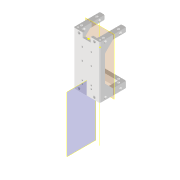
# Autodesk Inventor part: 30_Linear_Stage_NEMA11_China_base_universal_v3
Saved by Autodesk Inventor 2022 (Build 260153000, 153)
## iProperties
Created: 2022-02-11
Part Number: 30_Linear_Stage_NEMA11_China_base_universal_v3
Material: Generic
Document SubType Name: Modeling
Designer: wanghaoran
Density: 1 g/cm^3
Appearance: Default
Catalog Web Link: isPrinted
Vendor: openUC2
Mass: 36.1859 g
Surface Area: 194.638 cm^2
Volume: 36.1859 cm^3
Author: wanghaoran
Autodesk Inventor part; units mm, degrees
note: some values were not read from the file. Chosen so that the rebuilt part matches the saved one: pattern direction of "Runde Anordnung2".
ref_plane "YZ Plane" through (0, 0, 0) normal (1, 0, 0) x (0, 1, 0)
ref_plane "XZ Plane" through (0, 0, 0) normal (0, 1, 0) x (-1, 0, 0)
sketch "Sketch1" plane through (0, 0, 0) normal (0, 1, 0) x (-1, 0, 0)
  line L0 (0, 0) -> (49.8, 0)
  line L1 (49.8, 0) -> (49.8, -49.8)
  line L2 (49.8, -49.8) -> (0, -49.8)
  line L3 (0, -49.8) -> (0, 0)
  line L4 (7.8, -7.8) -> (42, -7.8)
  line L5 (42, -7.8) -> (42, -42)
  line L6 (42, -42) -> (7.8, -42)
  line L7 (7.8, -42) -> (7.8, -7.8)
  line L8 (39.9, -4.55) -> (9.9, -4.55) projected
  line L9 (42, -7.8) -> (7.8, -7.8)
  line L10 (7.8, -7.8) -> (7.8, -4.55)
  line L11 (7.8, -4.55) -> (42, -4.55)
  line L12 (42, -4.55) -> (42, -7.8)
  dimension "d0" = 49.8
  dimension "d1" = 49.8
  dimension "d2" = 7.8
  constraints: 24 end point, 6 parallel, 3 perpendicular, 2 horizontal, 3 other
  measures "d0" distance of L1.end L2.end
  measures "d1" distance of L0.end L1.end
  measures "d2" distance between parallel lines of L3 L7
extrude "Extrusion1" add sketch "Sketch1" along normal blind 12
sketch "Sketch3" plane through (0, 0, 0) normal (0, -1, 0) x (1, 0, 0)
  line L0 (-49.8, 0) -> (0, 0) projected
  line L1 (-49.8, -49.8) -> (-49.8, 0) projected
  line L2 (0, 0) -> (-49.8, 0)
  line L3 (-49.8, 0) -> (-49.8, -4.55)
  line L4 (-49.8, -4.55) -> (0, -4.55)
  line L5 (0, -4.55) -> (0, 0)
  line L6 (-7.8, -42) -> (-7.8, -4.55) projected
  line L7 (0, -49.8) -> (-7.8, -49.8)
  line L8 (-7.8, -49.8) -> (-7.8, -42)
  line L9 (-7.8, -42) -> (0, -42)
  line L10 (0, -42) -> (0, -49.8)
  line L11 (0, -49.8) -> (-49.8, -49.8) projected
  line L12 (-42, -4.55) -> (-42, -42) projected
  line L13 (-49.8, -49.8) -> (-42, -49.8)
  line L14 (-42, -49.8) -> (-42, -42)
  line L15 (-42, -42) -> (-49.8, -42)
  line L16 (-49.8, -42) -> (-49.8, -49.8)
  line L17 (-7.8, -4.55) -> (-42, -4.55) projected
  line L18 (-49.8, -4.55) -> (-42, -4.55)
  line L19 (-42, -4.55) -> (-42, -10)
  line L20 (-42, -10) -> (-49.8, -10)
  line L21 (-49.8, -10) -> (-49.8, -4.55)
  line L22 (0, -4.55) -> (-7.8, -4.55)
  line L23 (-7.8, -4.55) -> (-7.8, -10)
  line L24 (-7.8, -10) -> (0, -10)
  line L25 (0, -10) -> (0, -4.55)
  point P0 (-7.8, -7.8)
  point P1 (-42, -7.8)
  point P2 (-7.8, -7.8)
  point P3 (-42, -7.8)
  dimension "d57" = 0
  dimension "d58" = 10
  dimension "d59" = 10
  constraints: 40 end point, 10 parallel, 5 horizontal, 5 perpendicular, 3 point on line
  measures "d57" distance between parallel lines of L17 L4
  measures "d58" distance between parallel lines of L20 L0
  measures "d59" distance between parallel lines of L24 L0
extrude "Extrusion2" add sketch "Sketch3" against normal blind 92 contours L0 L5 L4 L1 | L4 L12 L20 L1 | L25 L24 L6 L4
sketch "Sketch4" plane through (-49.8, 0, 0) normal (0, 0, 1) x (1, 0, 0)
  line L0 (23.45, 81) -> (26.35, 81)
  line L1 (26.35, 81) -> (26.35, 11)
  line L2 (26.35, 11) -> (23.45, 11)
  line L3 (23.45, 11) -> (23.45, 81)
  line L4 (49.8, 0) -> (49.8, 92) projected
  line L5 (0, 0) -> (49.8, 0) projected
  circle A0 centre (24.9, 81) radius 1.45
  circle A1 centre (24.9, 11) radius 1.45
  line L6 (0, 92) -> (49.8, 92) projected
  circle A2 centre (33.4, 21) radius 1.45
  circle A3 centre (16.4, 21) radius 1.45
  circle A4 centre (33.4, 76) radius 1.45
  circle A5 centre (16.4, 76) radius 1.45
  line L7 (-75.7089, 93.7838) -> (-35.7089, 93.7838)
  line L8 (-35.7089, 93.7838) -> (-35.7089, -0.2162)
  line L9 (-35.7089, -0.2162) -> (-75.7089, -0.2162)
  line L10 (-75.7089, -0.2162) -> (-75.7089, 93.7838)
  circle A6 centre (-67.7652, 52.7838) radius 1.45
  circle A7 centre (-67.7652, 14.7838) radius 1.45
  circle A8 centre (16.4, 15) radius 1.45
  circle A9 centre (33.4, 15) radius 1.45
  circle A10 centre (16.4, 53) radius 1.45
  circle A11 centre (33.4, 53) radius 1.45
  dimension "d9" = 2.9
  dimension "d10" = 70
  dimension "d11" = 23.45
  dimension "d12" = 11
  dimension "d123" = 2.9
  dimension "d125" = 21
  dimension "d128" = 7.05
  dimension "d131" = 17
  dimension "d134" = 55
  dimension "d155" = 40
  dimension "d156" = 94
  dimension "d157" = 2.9
  dimension "d161" = 38
  dimension "d166" = 15
  dimension "d167" = 2.9
  dimension "d168" = 2.9
  dimension "d169" = 15
  dimension "d170" = 15
  dimension "d173" = 38
  constraints: 16 end point, 10 centre point, 4 parallel, 3 horizontal, 3 vertical, 2 midpoint, 2 perpendicular, 18 other
  measures "d9" distance of L1.end L2.end
  measures "d10" distance of L0.end L1.end
  measures "d11" distance between parallel lines of L4 L1
  measures "d12" distance between parallel lines of L5 L2
  measures "d123" diameter of A2
  measures "d125" distance from line of L5 A2.centre
  measures "d128" distance from line of A2.centre L1
  measures "d131" distance of A2.centre A3.centre
  measures "d134" distance of A2.centre A4.centre
  measures "d155" distance of L8.end L9.end
  measures "d156" distance of L7.end L8.end
  measures "d157" diameter of A6
  measures "d161" distance of A6.centre A7.centre
  measures "d166" distance from line of L9 A7.centre
  measures "d167" diameter of A8
  measures "d168" diameter of A9
  measures "d169" distance from line of L5 A8.centre
  measures "d170" distance from line of L5 A9.centre
  measures "d173" distance of A8.centre A10.centre
extrude "Extrusion3" cut sketch "Sketch4" against normal up to next contours A2 | A3 | A4 | A5 | A8 | A9 | A10 | A11
sketch "Sketch5" plane through (0, 92, 0) normal (0, 1, 0) x (1, 0, 0)
  circle A0 centre (-45.9, 45.9) radius 1.4
  circle A1 centre (-3.9, 45.9) radius 1.4
  line L0 (-49.8, 49.8) -> (-49.8, 0) projected
  line L1 (-49.8, 24.9) -> (-42, 24.9)
  line L2 (-42, 4.55) -> (-42, 42) projected
  line L3 (-49.8, 0) -> (0, 0) projected
  line L4 (0, 0) -> (0, 10) projected
  line L5 (0, 10) -> (-7.8, 10) projected
  line L6 (-7.8, 10) -> (-7.8, 4.55) projected
  line L7 (-49.8, 10) -> (-49.8, 0) projected
  line L8 (0, 49.8) -> (-49.8, 49.8) projected
  line L9 (-49.8, 0) -> (0, 0)
  line L10 (0, 0) -> (0, 49.8)
  line L11 (0, 49.8) -> (-49.8, 49.8)
  line L12 (-49.8, 49.8) -> (-49.8, 0)
  circle A2 centre (-4.9, 4.9) radius 2.4
  circle A3 centre (-44.9, 4.9) radius 2.4
  circle A4 centre (-4.9, 4.9) radius 1.4
  circle A5 centre (-44.9, 4.9) radius 1.4
  line L13 (-7.8, 4.55) -> (-42, 4.55) projected
  line L14 (-42, 4.55) -> (-42, 10) projected
  line L15 (-42, 10) -> (-49.8, 10) projected
  point P0 (-42, 7.8)
  dimension "d28" = 2.8
  dimension "d29" = 2.8
  dimension "d90" = 2.8
  dimension "d91" = 2.8
  dimension "d92" = 40
  dimension "d93" = 4.9
  dimension "d94" = 4.9
  dimension "d95" = 4.9
  constraints: 10 end point, 6 centre point, 2 coincident, 2 horizontal, 2 parallel, 1 midpoint, 1 perpendicular, 1 point on line
  measures "d28" diameter of A0
  measures "d29" diameter of A1
  measures "d90" diameter of A4
  measures "d91" diameter of A5
  measures "d92" distance of A4.centre A5.centre
  measures "d93" distance from line of L12 A5.centre
  measures "d94" distance from line of L3 A5.centre
  measures "d95" distance from line of L9 A2.centre
extrude "Extrusion4" cut sketch "Sketch5" against normal blind 20 contours A0 | A1 | A4 | A5
fillet "Fillet1" radius 2 4 edges at (0, 46, 0) (0, 6, -49.8) (-49.8, 6, -49.8) (-49.8, 46, 0)
ref_plane "Arbeitsebene1" through (-24.9, 12, -4.55) normal (-1, 0, 0) x (0, 0, -1)
ref_plane "Arbeitsebene2" through (-47.8, 0, -24.9) normal (0, 0, 1) x (1, 0, 0)
sketch "Skizze8" plane through (0, 0, 0) normal (0, -1, 0) x (1, 0, 0)
  line L0 (-49.9, -29.9) -> (-49.9, -47.9) projected
  arc A0 (-49.9, -47.9) -> (-47.9, -49.9) centre (-47.9, -47.9) ccw projected
  line L1 (-30.0511, -49.9) -> (-47.9, -49.9) projected
  line L2 (-30.0511, -49.9) -> (-30.0509, -49.1742) projected
  arc A1 (-30.0509, -49.1742) -> (-30.2806, -48.8498) centre (-30.3999, -49.1778) ccw projected
  arc A2 (-31.9947, -46.7407) -> (-30.2806, -48.8498) centre (-29.84, -46.7407) ccw projected
  line L3 (-31.9947, -46.7407) -> (-31.9947, -46.6009) projected
  arc A3 (-29.8434, -44.4498) -> (-31.9947, -46.6009) centre (-29.8435, -46.6009) ccw projected
  line L4 (-29.8434, -44.4498) -> (-19.9598, -44.4503) projected
  arc A4 (-17.81, -46.6004) -> (-19.9598, -44.4503) centre (-19.96, -46.6003) ccw projected
  line L5 (-17.81, -46.6004) -> (-17.81, -46.7408) projected
  arc A5 (-19.52, -48.8451) -> (-17.81, -46.7408) centre (-19.9599, -46.7406) ccw projected
  arc A6 (-19.52, -48.8451) -> (-19.7498, -49.1739) centre (-19.3996, -49.1739) ccw projected
  line L6 (-19.7498, -49.1739) -> (-19.7495, -49.9) projected
  line L7 (-1.9, -49.9) -> (-19.7495, -49.9) projected
  arc A7 (-1.9, -49.9) -> (0.1, -47.9) centre (-1.9, -47.9) ccw projected
  line L8 (0.1, -47.9) -> (0.1, -30.0511) projected
  line L9 (0.1, -30.0511) -> (-0.6258, -30.0509) projected
  arc A8 (-0.6258, -30.0509) -> (-0.9502, -30.2806) centre (-0.6222, -30.3999) ccw projected
  arc A9 (-3.0593, -31.9947) -> (-0.9502, -30.2806) centre (-3.0593, -29.84) ccw projected
  line L10 (-3.0593, -31.9947) -> (-3.1991, -31.9947) projected
  arc A10 (-5.3502, -29.8434) -> (-3.1991, -31.9947) centre (-3.1991, -29.8435) ccw projected
  line L11 (-5.3502, -29.8434) -> (-5.3497, -19.9598) projected
  arc A11 (-3.1996, -17.81) -> (-5.3497, -19.9598) centre (-3.1997, -19.96) ccw projected
  line L12 (-3.1996, -17.81) -> (-3.0592, -17.81) projected
  arc A12 (-0.9549, -19.52) -> (-3.0592, -17.81) centre (-3.0594, -19.9599) ccw projected
  arc A13 (-0.9549, -19.52) -> (-0.6261, -19.7498) centre (-0.6261, -19.3996) ccw projected
  line L13 (-0.6261, -19.7498) -> (0.1, -19.7495) projected
  line L14 (0.1, -19.7495) -> (0.1, -1.9) projected
  arc A14 (0.1, -1.9) -> (-1.9, 0.1) centre (-1.9, -1.9) ccw projected
  line L15 (-19.9, 0.1) -> (-1.9, 0.1) projected
  line L16 (-19.9, 0.1) -> (-19.9, 0.9263) projected
  arc A15 (-19.56, 1.4) -> (-19.9, 0.9263) centre (-19.4, 0.9263) ccw projected
  arc A16 (-19.56, 1.4) -> (-17.96, 3.3596) centre (-19.96, 3.3596) ccw projected
  line L17 (-17.96, 3.3596) -> (-17.96, 3.5) projected
  arc A17 (-17.96, 3.5) -> (-19.96, 5.5) centre (-19.96, 3.5) ccw projected
  line L18 (-19.96, 5.5) -> (-29.84, 5.5) projected
  arc A18 (-29.84, 5.5) -> (-31.84, 3.5) centre (-29.84, 3.5) ccw projected
  line L19 (-31.84, 3.5) -> (-31.84, 3.3596) projected
  arc A19 (-31.84, 3.3596) -> (-30.24, 1.4) centre (-29.84, 3.3596) ccw projected
  arc A20 (-29.9, 0.9263) -> (-30.24, 1.4) centre (-30.4, 0.9263) ccw projected
  line L20 (-29.9, 0.9263) -> (-29.9, 0.1) projected
  line L21 (-47.9, 0.1) -> (-29.9, 0.1) projected
  arc A21 (-47.9, 0.1) -> (-49.9, -1.9) centre (-47.9, -1.9) ccw projected
  line L22 (-49.9, -1.9) -> (-49.9, -19.9) projected
  line L23 (-49.9, -19.9) -> (-50.7263, -19.9) projected
  arc A22 (-51.2, -19.56) -> (-50.7263, -19.9) centre (-50.7263, -19.4) ccw projected
  arc A23 (-51.2, -19.56) -> (-53.1596, -17.96) centre (-53.1596, -19.96) ccw projected
  line L24 (-53.1596, -17.96) -> (-53.3, -17.96) projected
  arc A24 (-53.3, -17.96) -> (-55.3, -19.96) centre (-53.3, -19.96) ccw projected
  line L25 (-55.3, -19.96) -> (-55.3, -29.84) projected
  arc A25 (-55.3, -29.84) -> (-53.3, -31.84) centre (-53.3, -29.84) ccw projected
  line L26 (-53.3, -31.84) -> (-53.1596, -31.84) projected
  arc A26 (-53.1596, -31.84) -> (-51.2, -30.24) centre (-53.1596, -29.84) ccw projected
  arc A27 (-50.7263, -29.9) -> (-51.2, -30.24) centre (-50.7263, -30.4) ccw projected
  line L27 (-50.7263, -29.9) -> (-49.9, -29.9) projected
  arc A28 (-49.9, -26.2329) -> (-49.9, -23.7671) centre (-46.2, -25) ccw projected
  line L28 (-49.9, -26.2329) -> (-49.9, -23.7671) projected
  circle A29 centre (-25, -3.6) radius 3.9 projected
  line L29 (-7.6, -40.2) -> (-7.6, -9.6) projected
  arc A30 (-9.6, -42.2) -> (-7.6, -40.2) centre (-9.6, -40.2) ccw projected
  line L30 (-9.6, -42.2) -> (-40.2, -42.2) projected
  arc A31 (-42.2, -40.2) -> (-40.2, -42.2) centre (-40.2, -40.2) ccw projected
  line L31 (-42.2, -9.6) -> (-42.2, -40.2) projected
  arc A32 (-40.2, -7.6) -> (-42.2, -9.6) centre (-40.2, -9.6) ccw projected
  line L32 (-40.2, -7.6) -> (-9.6, -7.6) projected
  arc A33 (-7.6, -9.6) -> (-9.6, -7.6) centre (-9.6, -9.6) ccw projected
  circle A34 centre (-44.8, -5) radius 2.4 projected
  circle A35 centre (-39.35, -4.35) radius 2.45 projected
  circle A36 centre (-45.45, -10.45) radius 2.45 projected
  circle A37 centre (-4.35, -10.45) radius 2.45 projected
  circle A38 centre (-10.45, -4.35) radius 2.45 projected
  circle A39 centre (-5, -5) radius 2.4 projected
  circle A40 centre (-45.45, -39.35) radius 2.45 projected
  circle A41 centre (-39.35, -45.45) radius 2.45 projected
  circle A42 centre (-44.8, -44.8) radius 2.4 projected
  circle A43 centre (-4.35, -39.35) radius 2.45 projected
  circle A44 centre (-10.45, -45.45) radius 2.45 projected
  circle A45 centre (-5, -44.8) radius 2.4 projected
  point P0 (0, 0)
hole "Bohrung1" at (-45.45, 0, -39.35) at (-39.35, 0, -4.35) at (-10.45, 0, -4.35) at (-4.35, 0, -39.35) at (-10.45, 0, -45.45) at (-39.35, 0, -45.45) direction (0, 1, 0) diameter 4.8 depth 12 tip angle 118
sketch "Skizze10" plane through (0, 92, 0) normal (0, 1, 0) x (1, 0, 0)
  arc A0 (-25.6984, 4.55) -> (-24.1016, 4.55) centre (-24.9, 3.4) ccw projected
  point P0 (0, 0)
sketch "Skizze11" plane through (-47.8, 0, 0) normal (0, 0, 1) x (1, 0, 0)
  line L0 (7.74, 57.65) -> (37.74, 57.65) projected
  arc A0 (5.24, 60.15) -> (7.74, 57.65) centre (7.74, 60.15) ccw projected
  line L1 (5.24, 90.15) -> (5.24, 60.15) projected
  arc A1 (7.74, 92.65) -> (5.24, 90.15) centre (7.74, 90.15) ccw projected
  line L2 (37.74, 92.65) -> (7.74, 92.65) projected
  arc A2 (40.24, 90.15) -> (37.74, 92.65) centre (37.74, 90.15) ccw projected
  line L3 (40.24, 60.15) -> (40.24, 90.15) projected
  arc A3 (37.74, 57.65) -> (40.24, 60.15) centre (37.74, 60.15) ccw projected
  circle A4 centre (22.74, 53.15) radius 4 projected
  line L4 (40.99, 91.1222) -> (43.54, 92.5945) projected
  line L5 (43.54, 92.5945) -> (46.09, 91.1222) projected
  line L6 (46.09, 91.1222) -> (46.09, 88.1778) projected
  line L7 (46.09, 88.1778) -> (43.54, 86.7055) projected
  line L8 (43.54, 86.7055) -> (40.99, 88.1778) projected
  line L9 (40.99, 88.1778) -> (40.99, 91.1222) projected
  line L10 (35.7678, 93.4) -> (34.2955, 95.95) projected
  line L11 (34.2955, 95.95) -> (35.7678, 98.5) projected
  line L12 (35.7678, 98.5) -> (38.7122, 98.5) projected
  line L13 (38.7122, 98.5) -> (40.1845, 95.95) projected
  line L14 (40.1845, 95.95) -> (38.7122, 93.4) projected
  line L15 (38.7122, 93.4) -> (35.7678, 93.4) projected
  line L16 (40.99, 59.1778) -> (43.54, 57.7055) projected
  line L17 (40.99, 62.1222) -> (40.99, 59.1778) projected
  line L18 (43.54, 63.5945) -> (40.99, 62.1222) projected
  line L19 (46.09, 62.1222) -> (43.54, 63.5945) projected
  line L20 (46.09, 59.1778) -> (46.09, 62.1222) projected
  line L21 (43.54, 57.7055) -> (46.09, 59.1778) projected
  line L22 (35.7678, 56.9) -> (34.2955, 54.35) projected
  line L23 (38.7122, 56.9) -> (35.7678, 56.9) projected
  line L24 (40.1845, 54.35) -> (38.7122, 56.9) projected
  line L25 (38.7122, 51.8) -> (40.1845, 54.35) projected
  line L26 (35.7678, 51.8) -> (38.7122, 51.8) projected
  line L27 (34.2955, 54.35) -> (35.7678, 51.8) projected
  line L28 (4.49, 91.1222) -> (1.94, 92.5945) projected
  line L29 (4.49, 88.1778) -> (4.49, 91.1222) projected
  line L30 (1.94, 86.7055) -> (4.49, 88.1778) projected
  line L31 (-0.61, 88.1778) -> (1.94, 86.7055) projected
  line L32 (-0.61, 91.1222) -> (-0.61, 88.1778) projected
  line L33 (1.94, 92.5945) -> (-0.61, 91.1222) projected
  line L34 (9.7122, 93.4) -> (11.1845, 95.95) projected
  line L35 (6.7678, 93.4) -> (9.7122, 93.4) projected
  line L36 (5.2955, 95.95) -> (6.7678, 93.4) projected
  line L37 (6.7678, 98.5) -> (5.2955, 95.95) projected
  line L38 (9.7122, 98.5) -> (6.7678, 98.5) projected
  line L39 (11.1845, 95.95) -> (9.7122, 98.5) projected
  line L40 (9.7122, 56.9) -> (11.1845, 54.35) projected
  line L41 (11.1845, 54.35) -> (9.7122, 51.8) projected
  line L42 (9.7122, 51.8) -> (6.7678, 51.8) projected
  line L43 (6.7678, 51.8) -> (5.2955, 54.35) projected
  line L44 (5.2955, 54.35) -> (6.7678, 56.9) projected
  line L45 (6.7678, 56.9) -> (9.7122, 56.9) projected
  line L46 (4.49, 59.1778) -> (1.94, 57.7055) projected
  line L47 (1.94, 57.7055) -> (-0.61, 59.1778) projected
  line L48 (-0.61, 59.1778) -> (-0.61, 62.1222) projected
  line L49 (-0.61, 62.1222) -> (1.94, 63.5945) projected
  line L50 (1.94, 63.5945) -> (4.49, 62.1222) projected
  line L51 (4.49, 62.1222) -> (4.49, 59.1778) projected
  circle A5 centre (0.74, 75.15) radius 4 projected
  line L52 (46.8233, 69.2502) -> (47.24, 69.2503) projected
  arc A6 (41.54, 70.1) -> (46.8233, 69.2502) centre (44.25, 70.1) ccw projected
  line L53 (41.54, 80.2) -> (41.54, 70.1) projected
  arc A7 (46.8233, 81.0498) -> (41.54, 80.2) centre (44.25, 80.2) ccw projected
  line L54 (47.24, 81.0497) -> (46.8233, 81.0498) projected
  line L55 (47.24, 98.15) -> (47.24, 81.0497) projected
  arc A8 (47.24, 98.15) -> (45.74, 99.65) centre (45.74, 98.15) ccw projected
  line L56 (28.6397, 99.65) -> (45.74, 99.65) projected
  line L57 (28.6398, 99.2333) -> (28.6397, 99.65) projected
  arc A9 (27.79, 93.95) -> (28.6398, 99.2333) centre (27.79, 96.66) ccw projected
  line L58 (17.69, 93.95) -> (27.79, 93.95) projected
  arc A10 (16.8402, 99.2333) -> (17.69, 93.95) centre (17.69, 96.66) ccw projected
  line L59 (16.8403, 99.65) -> (16.8402, 99.2333) projected
  line L60 (-0.26, 99.65) -> (16.8403, 99.65) projected
  arc A11 (-0.26, 99.65) -> (-1.76, 98.15) centre (-0.26, 98.15) ccw projected
  line L61 (-1.76, 79.65) -> (-1.76, 98.15) projected
  line L62 (-3.6239, 79.65) -> (-1.76, 79.65) projected
  arc A12 (-4.3693, 80.3167) -> (-3.6239, 79.65) centre (-3.6239, 80.4) ccw projected
  arc A13 (-4.3693, 80.3167) -> (-7.36, 80.15) centre (-5.86, 80.15) ccw projected
  line L63 (-7.36, 70.15) -> (-7.36, 80.15) projected
  arc A14 (-7.36, 70.15) -> (-4.3693, 69.9833) centre (-5.86, 70.15) ccw projected
  arc A15 (-3.6239, 70.65) -> (-4.3693, 69.9833) centre (-3.6239, 69.9) ccw projected
  line L64 (-1.76, 70.65) -> (-3.6239, 70.65) projected
  line L65 (-1.76, 52.15) -> (-1.76, 70.65) projected
  arc A16 (-1.76, 52.15) -> (-0.26, 50.65) centre (-0.26, 52.15) ccw projected
  line L66 (18.24, 50.65) -> (-0.26, 50.65) projected
  line L67 (18.24, 48.7861) -> (18.24, 50.65) projected
  arc A17 (17.5733, 48.0407) -> (18.24, 48.7861) centre (17.49, 48.7861) ccw projected
  arc A18 (17.5733, 48.0407) -> (17.74, 45.05) centre (17.74, 46.55) ccw projected
  line L68 (27.74, 45.05) -> (17.74, 45.05) projected
  arc A19 (27.74, 45.05) -> (27.9067, 48.0407) centre (27.74, 46.55) ccw projected
  arc A20 (27.24, 48.7861) -> (27.9067, 48.0407) centre (27.99, 48.7861) ccw projected
  line L69 (27.24, 50.65) -> (27.24, 48.7861) projected
  line L70 (45.74, 50.65) -> (27.24, 50.65) projected
  arc A21 (45.74, 50.65) -> (47.24, 52.15) centre (45.74, 52.15) ccw projected
  line L71 (47.24, 69.2503) -> (47.24, 52.15) projected
  line L72 (7.74, 7.65) -> (37.74, 7.65) projected
  arc A22 (5.24, 10.15) -> (7.74, 7.65) centre (7.74, 10.15) ccw projected
  line L73 (5.24, 40.15) -> (5.24, 10.15) projected
  arc A23 (7.74, 42.65) -> (5.24, 40.15) centre (7.74, 40.15) ccw projected
  line L74 (37.74, 42.65) -> (7.74, 42.65) projected
  arc A24 (40.24, 40.15) -> (37.74, 42.65) centre (37.74, 40.15) ccw projected
  line L75 (40.24, 10.15) -> (40.24, 40.15) projected
  arc A25 (37.74, 7.65) -> (40.24, 10.15) centre (37.74, 10.15) ccw projected
  circle A26 centre (22.74, 3.15) radius 4 projected
  line L76 (40.99, 41.1222) -> (43.54, 42.5945) projected
  line L77 (43.54, 42.5945) -> (46.09, 41.1222) projected
  line L78 (46.09, 41.1222) -> (46.09, 38.1778) projected
  line L79 (46.09, 38.1778) -> (43.54, 36.7055) projected
  line L80 (43.54, 36.7055) -> (40.99, 38.1778) projected
  line L81 (40.99, 38.1778) -> (40.99, 41.1222) projected
  line L82 (35.7678, 43.4) -> (34.2955, 45.95) projected
  line L83 (34.2955, 45.95) -> (35.7678, 48.5) projected
  line L84 (35.7678, 48.5) -> (38.7122, 48.5) projected
  line L85 (38.7122, 48.5) -> (40.1845, 45.95) projected
  line L86 (40.1845, 45.95) -> (38.7122, 43.4) projected
  line L87 (38.7122, 43.4) -> (35.7678, 43.4) projected
  line L88 (40.99, 9.1778) -> (43.54, 7.7055) projected
  line L89 (40.99, 12.1222) -> (40.99, 9.1778) projected
  line L90 (43.54, 13.5945) -> (40.99, 12.1222) projected
  line L91 (46.09, 12.1222) -> (43.54, 13.5945) projected
  line L92 (46.09, 9.1778) -> (46.09, 12.1222) projected
  line L93 (43.54, 7.7055) -> (46.09, 9.1778) projected
  line L94 (35.7678, 6.9) -> (34.2955, 4.35) projected
  line L95 (38.7122, 6.9) -> (35.7678, 6.9) projected
  line L96 (40.1845, 4.35) -> (38.7122, 6.9) projected
  line L97 (38.7122, 1.8) -> (40.1845, 4.35) projected
  line L98 (35.7678, 1.8) -> (38.7122, 1.8) projected
  line L99 (34.2955, 4.35) -> (35.7678, 1.8) projected
  line L100 (4.49, 41.1222) -> (1.94, 42.5945) projected
  line L101 (4.49, 38.1778) -> (4.49, 41.1222) projected
  line L102 (1.94, 36.7055) -> (4.49, 38.1778) projected
  line L103 (-0.61, 38.1778) -> (1.94, 36.7055) projected
  line L104 (-0.61, 41.1222) -> (-0.61, 38.1778) projected
  line L105 (1.94, 42.5945) -> (-0.61, 41.1222) projected
  line L106 (9.7122, 43.4) -> (11.1845, 45.95) projected
  line L107 (6.7678, 43.4) -> (9.7122, 43.4) projected
  line L108 (5.2955, 45.95) -> (6.7678, 43.4) projected
  line L109 (6.7678, 48.5) -> (5.2955, 45.95) projected
  line L110 (9.7122, 48.5) -> (6.7678, 48.5) projected
  line L111 (11.1845, 45.95) -> (9.7122, 48.5) projected
  line L112 (9.7122, 6.9) -> (11.1845, 4.35) projected
  line L113 (11.1845, 4.35) -> (9.7122, 1.8) projected
  line L114 (9.7122, 1.8) -> (6.7678, 1.8) projected
  line L115 (6.7678, 1.8) -> (5.2955, 4.35) projected
  line L116 (5.2955, 4.35) -> (6.7678, 6.9) projected
  line L117 (6.7678, 6.9) -> (9.7122, 6.9) projected
  line L118 (4.49, 9.1778) -> (1.94, 7.7055) projected
  line L119 (1.94, 7.7055) -> (-0.61, 9.1778) projected
  line L120 (-0.61, 9.1778) -> (-0.61, 12.1222) projected
  line L121 (-0.61, 12.1222) -> (1.94, 13.5945) projected
  line L122 (1.94, 13.5945) -> (4.49, 12.1222) projected
  line L123 (4.49, 12.1222) -> (4.49, 9.1778) projected
  circle A27 centre (0.74, 25.15) radius 4 projected
  line L124 (46.8233, 19.2502) -> (47.24, 19.2503) projected
  arc A28 (41.54, 20.1) -> (46.8233, 19.2502) centre (44.25, 20.1) ccw projected
  line L125 (41.54, 30.2) -> (41.54, 20.1) projected
  arc A29 (46.8233, 31.0498) -> (41.54, 30.2) centre (44.25, 30.2) ccw projected
  line L126 (47.24, 31.0497) -> (46.8233, 31.0498) projected
  line L127 (47.24, 48.15) -> (47.24, 31.0497) projected
  arc A30 (47.24, 48.15) -> (45.74, 49.65) centre (45.74, 48.15) ccw projected
  line L128 (28.6397, 49.65) -> (45.74, 49.65) projected
  line L129 (28.6398, 49.2333) -> (28.6397, 49.65) projected
  arc A31 (27.79, 43.95) -> (28.6398, 49.2333) centre (27.79, 46.66) ccw projected
  line L130 (17.69, 43.95) -> (27.79, 43.95) projected
  arc A32 (16.8402, 49.2333) -> (17.69, 43.95) centre (17.69, 46.66) ccw projected
  line L131 (16.8403, 49.65) -> (16.8402, 49.2333) projected
  line L132 (-0.26, 49.65) -> (16.8403, 49.65) projected
  arc A33 (-0.26, 49.65) -> (-1.76, 48.15) centre (-0.26, 48.15) ccw projected
  line L133 (-1.76, 29.65) -> (-1.76, 48.15) projected
  line L134 (-3.6239, 29.65) -> (-1.76, 29.65) projected
  arc A34 (-4.3693, 30.3167) -> (-3.6239, 29.65) centre (-3.6239, 30.4) ccw projected
  arc A35 (-4.3693, 30.3167) -> (-7.36, 30.15) centre (-5.86, 30.15) ccw projected
  line L135 (-7.36, 20.15) -> (-7.36, 30.15) projected
  arc A36 (-7.36, 20.15) -> (-4.3693, 19.9833) centre (-5.86, 20.15) ccw projected
  arc A37 (-3.6239, 20.65) -> (-4.3693, 19.9833) centre (-3.6239, 19.9) ccw projected
  line L136 (-1.76, 20.65) -> (-3.6239, 20.65) projected
  line L137 (-1.76, 2.15) -> (-1.76, 20.65) projected
  arc A38 (-1.76, 2.15) -> (-0.26, 0.65) centre (-0.26, 2.15) ccw projected
  line L138 (18.24, 0.65) -> (-0.26, 0.65) projected
  line L139 (18.24, -1.2139) -> (18.24, 0.65) projected
  arc A39 (17.5733, -1.9593) -> (18.24, -1.2139) centre (17.49, -1.2139) ccw projected
  arc A40 (17.5733, -1.9593) -> (17.74, -4.95) centre (17.74, -3.45) ccw projected
  line L140 (27.74, -4.95) -> (17.74, -4.95) projected
  arc A41 (27.74, -4.95) -> (27.9067, -1.9593) centre (27.74, -3.45) ccw projected
  arc A42 (27.24, -1.2139) -> (27.9067, -1.9593) centre (27.99, -1.2139) ccw projected
  line L141 (27.24, 0.65) -> (27.24, -1.2139) projected
  line L142 (45.74, 0.65) -> (27.24, 0.65) projected
  arc A43 (45.74, 0.65) -> (47.24, 2.15) centre (45.74, 2.15) ccw projected
  line L143 (47.24, 19.2503) -> (47.24, 2.15) projected
  point P0 (1.94, 60.65)
  point P1 (43.54, 60.65)
  point P2 (-0.26, 50.15)
  point P3 (45.74, 50.15)
  point P4 (8.24, 4.35)
  point P5 (1.94, 39.65)
  point P6 (37.24, 4.35)
  point P7 (43.54, 39.65)
hole "Bohrung3" at (-39.56, 4.35, 0) at (-10.56, 4.35, 0) direction (0, 0, -1) diameter 4.8 depth 12 tip angle 118
pattern_circular "Runde Anordnung1" count 4 over 360 about axis through (-24.9, -3.9, -24.9) along (0, -1, 0) of "Bohrung3"
sketch "Skizze14" plane through (0, 92, 0) normal (0, 1, 0) x (1, 0, 0)
  circle A0 centre (-10.45, 45.45) radius 2.3 projected
  circle A1 centre (-4.35, 10.45) radius 2.3 projected
  circle A2 centre (-45.45, 39.35) radius 2.3 projected
  circle A3 centre (-45.45, 10.45) radius 2.3 projected
  circle A4 centre (-4.35, 39.35) radius 2.3 projected
  circle A5 centre (-39.35, 45.45) radius 2.3 projected
  line L0 (-9.3, 42) -> (-40.5, 42) projected
  line L1 (-9.3, 7.8) -> (-9.3, 42) projected
  line L2 (-9.7, 7.8) -> (-9.3, 7.8) projected
  line L3 (-9.7, 4.35) -> (-9.7, 7.8) projected
  line L4 (-12.75, 4.35) -> (-9.7, 4.35) projected
  arc A6 (-12.7413, 4.55) -> (-12.75, 4.35) centre (-10.45, 4.35) ccw projected
  line L5 (-37.0587, 4.55) -> (-12.7413, 4.55) projected
  arc A7 (-37.05, 4.35) -> (-37.0587, 4.55) centre (-39.35, 4.35) ccw projected
  line L6 (-40.1, 4.35) -> (-37.05, 4.35) projected
  line L7 (-40.1, 7.8) -> (-40.1, 4.35) projected
  line L8 (-40.5, 7.8) -> (-40.1, 7.8) projected
  line L9 (-40.5, 42) -> (-40.5, 7.8) projected
  line L10 (-47.8, 49.8) -> (-2, 49.8) projected
  arc A8 (-47.8, 49.8) -> (-49.8, 47.8) centre (-47.8, 47.8) ccw projected
  line L11 (-49.8, 2) -> (-49.8, 47.8) projected
  arc A9 (-49.8, 2) -> (-47.8, 0) centre (-47.8, 2) ccw projected
  line L12 (-2, 0) -> (-47.8, 0) projected
  arc A10 (-2, 0) -> (0, 2) centre (-2, 2) ccw projected
  line L13 (0, 47.8) -> (0, 2) projected
  arc A11 (0, 47.8) -> (-2, 49.8) centre (-2, 47.8) ccw projected
  line L14 (-2, 49.8) -> (-47.8, 49.8) projected
  line L15 (-7.8, 42) -> (-7.8, 10) projected
  arc A12 (-47.8, 49.8) -> (-49.8, 47.8) centre (-47.8, 47.8) ccw projected
  arc A13 (0, 47.8) -> (-2, 49.8) centre (-2, 47.8) ccw projected
  arc A14 (-40.5, 47.75) -> (-42.4975, 49.8) centre (-42.4975, 47.8018) ccw
  line L16 (-40.5, 47.75) -> (-42.4975, 49.8) construction
  line L17 (-40.5, 47.75) -> (-37.6377, 47.75) construction
  arc A15 (-7.25, 49.8) -> (-9.3, 47.75) centre (-7.25, 47.75) ccw
  line L18 (-9.3, 47.75) -> (-7.25, 49.8) construction
  line L19 (-9.3, 47.75) -> (-6.4009, 47.75) construction
  line L20 (-42, 10) -> (-42, 42) projected
  line L21 (-40.5, 42) -> (-40.5, 49.8)
  line L22 (-9.3, 42) -> (-9.3, 49.8)
  point P0 (0, 0)
  point P1 (-7.25, 49.8)
  dimension "d121" = 134.257
  dimension "d122" = 45
  constraints: 12 end point, 6 point on line, 4 point on circle, 2 centre point, 2 equal length, 2 horizontal, 2 perpendicular, 2 tangent
  measures "d121" angle of L17 L16
  measures "d122" angle of L19 L18
ref_plane "Arbeitsebene3" through (-49.8, 100, -49.8) normal (0, -1, 0) x (1, 0, 0)
extrude "Extrusion7" add sketch "Skizze14" along normal up to surface (8 mm away) contours A0 L22 | A0 L22 A15 L10 A11 L13 A10 L12 A9 L11 A8 A14 L21 A5 L9 L8 L7 L6 A7 L5 A6 L4 L3 L2 L1 | A5 L21 picked at (-9.1703, 46.0197) picked at (-40.8781, 45.361)
sketch "Skizze15" plane through (-49.8, 0, 0) normal (0, 0, 1) x (1, 0, 0)
  circle A0 centre (39.24, 95.65) radius 2.45
  circle A1 centre (10.24, 95.65) radius 2.45
  circle A2 centre (10.24, 4.35) radius 2.4 projected
  circle A3 centre (39.24, 4.35) radius 2.4 projected
  line L0 (2, 0) -> (2, 100) projected
  line L1 (47.8, 100) -> (47.8, 0) projected
  line L2 (2, 100) -> (47.8, 100) projected
  line L3 (0, 100) -> (0, 0) projected
  line L4 (49.8, 0) -> (49.8, 100) projected
  point P0 (2, 41.0629)
  point P1 (2, 59.2371)
  point P2 (47.8, 59.8423)
  point P3 (47.8, 40.4577)
  point P4 (0, 61.4577)
  point P5 (49.8, 62.0629)
  dimension "d178" = 4.35
  dimension "d179" = 4.35
  dimension "d180" = 10.24
  dimension "d181" = 10.56
  constraints: 2 centre point
  measures "d178" distance from line of L2 A1.centre
  measures "d179" distance from line of L2 A0.centre
  measures "d180" distance from line of L3 A1.centre
  measures "d181" distance from line of L4 A0.centre
extrude "Extrusion8" cut sketch "Skizze15" against normal blind 10 contours A0 | A1
pattern_circular "Runde Anordnung2" count 3 over 180 about axis through (-24.9, -3.9, -24.9) along (0, -1, 0) of "Extrusion8" both ways yes
sketch "Skizze16" plane through (0, 0, -2) normal (1, 0, 0) x (0, 0, -1)
  line L0 (0, 0) -> (0, 100) projected
  line L1 (0, 0) -> (45.8, 0) projected
  line L2 (45.8, 12) -> (45.8, 0) projected
  line L3 (8, 12) -> (45.8, 12) projected
  line L4 (8, 12) -> (8, 92) projected
  line L5 (8, 92) -> (45.8, 92) projected
  line L6 (45.8, 92) -> (45.8, 100) projected
  line L7 (0, 100) -> (45.8, 100) projected
  circle A0 centre (8.24, 4.35) radius 2.4 projected
  circle A1 centre (37.24, 4.35) radius 2.4 projected
  line L8 (45.8, 92) -> (8, 92) projected
  line L9 (22.9, 92) -> (8, 77.1)
  line L10 (8, 12) -> (8, 92) projected
  line L11 (22.9, 92) -> (43.9718, 92) construction
  line L12 (40, 12) -> (8, 12) projected
  line L13 (22.9, 12) -> (8, 26.9)
  line L14 (22.9, 12) -> (43.9718, 12) construction
  point P0 (-2, 0)
  point P1 (8, 26.9)
  dimension "d109" = 135
  dimension "d110" = 135
  constraints: 8 end point, 4 point on line, 2 equal length, 2 horizontal
  measures "d109" angle of L9 L11
  measures "d110" angle of L14 L13
extrude "Extrusion9" add sketch "Skizze16" against normal up to surface (7.8 mm away) contours L9 L4 L5 | L3 L4 L13
mirror "Spiegeln2" about plane through (-24.9, 12, -4.55) normal (-1, 0, 0) of "Extrusion9"
sketch "Skizze17" plane through (-47.8, 100, 0) normal (0, 1, 0) x (1, 0, 0)
  line L0 (38.5, 47.75) -> (38.5, 7.8) projected
  line L1 (38.5, 7.8) -> (38.1, 7.8) projected
  line L2 (38.1, 7.8) -> (38.1, 4.35) projected
  line L3 (38.1, 4.35) -> (35.05, 4.35) projected
  arc A0 (35.0587, 4.55) -> (35.05, 4.35) centre (37.35, 4.35) ccw projected
  line L4 (35.0587, 4.55) -> (10.7413, 4.55) projected
  arc A1 (10.75, 4.35) -> (10.7413, 4.55) centre (8.45, 4.35) ccw projected
  line L5 (10.75, 4.35) -> (7.7, 4.35) projected
  line L6 (7.7, 4.35) -> (7.7, 7.8) projected
  line L7 (7.7, 7.8) -> (7.3, 7.8) projected
  line L8 (7.3, 7.8) -> (7.3, 47.75) projected
  circle A2 centre (43.45, 39.35) radius 2.3 projected
  circle A3 centre (2.35, 10.45) radius 2.3 projected
  circle A4 centre (2.35, 39.35) radius 2.3 projected
  circle A5 centre (43.45, 10.45) radius 2.3 projected
  arc A6 (-2, 2) -> (0, 0) centre (0, 2) ccw projected
  line L9 (0, 0) -> (45.8, 0) projected
  arc A7 (45.8, 0) -> (47.8, 2) centre (45.8, 2) ccw projected
  line L10 (47.8, 2) -> (47.8, 47.8) projected
  arc A8 (47.8, 47.8) -> (45.8, 49.8) centre (45.8, 47.8) ccw projected
  line L11 (5.3025, 49.8) -> (0, 49.8) projected
  arc A9 (0, 49.8) -> (-2, 47.8) centre (0, 47.8) ccw projected
  line L12 (-2, 47.8) -> (-2, 2) projected
  line L13 (5.8, 24.9) -> (-2, 24.9) projected
  circle A10 centre (2.35, 24.9) radius 1.4
  line L14 (47.8, 24.9) -> (40, 24.9) projected
  circle A11 centre (43.45, 24.9) radius 1.4
  arc A12 (7.3, 47.75) -> (5.3025, 49.8) centre (5.3025, 47.8018) ccw projected
  line L15 (45.8, 49.8) -> (40.55, 49.8) projected
  arc A13 (40.55, 49.8) -> (38.5, 47.75) centre (40.55, 47.75) ccw projected
  point P0 (47.8, 0)
  dimension "d113" = 2.8
  dimension "d114" = 2.8
  constraints: 2 centre point, 2 point on line
  measures "d113" diameter of A10
  measures "d114" diameter of A11
extrude "Extrusion10" cut sketch "Skizze17" against normal blind 10 contours A10 L13 | L13 A10 | A11 L14 | L14 A11
sketch "Sketch19" plane through (-47.8, 0, 0) normal (0, 0, 1) x (1, 0, 0)
  line L0 (15.4, 109) -> (30.4, 109)
  line L1 (30.4, 109) -> (30.4, 91)
  line L2 (30.4, 91) -> (15.4, 91)
  line L3 (15.4, 91) -> (15.4, 109)
  line L4 (0, 100) -> (45.8, 100) projected
  line L5 (15.4, 109) -> (30.4, 91) construction
  line L6 (30.4, 109) -> (15.4, 91) construction
  point P0 (47.8, 0)
  point P1 (22.9, 100)
  point P2 (30.4, 100)
  point P3 (15.4, 100)
  dimension "d151" = 15
  dimension "d152" = 18
  constraints: 12 end point, 3 midpoint, 2 parallel, 1 horizontal, 1 perpendicular
  measures "d151" distance of L1.end L2.end
  measures "d152" distance of L0.end L1.end
extrude "Extrusion12" cut sketch "Sketch19" against normal blind 10 contours L4 L1 L2 L3
sketch "Skizze20" plane through (0, 0, 0) normal (0, -1, 0) x (1, 0, 0)
  arc A0 (-36.9583, -4.55) -> (-41.7417, -4.55) centre (-39.35, -4.35) ccw projected
  line L0 (-12.8417, -4.55) -> (-36.9583, -4.55) projected
  arc A1 (-8.0583, -4.55) -> (-12.8417, -4.55) centre (-10.45, -4.35) ccw projected
  line L1 (-7.8, -4.55) -> (-8.0583, -4.55) projected
  line L2 (-7.8, -42) -> (-7.8, -4.55) projected
  line L3 (-42, -42) -> (-7.8, -42) projected
  line L4 (-42, -4.55) -> (-42, -42) projected
  line L5 (-41.7417, -4.55) -> (-42, -4.55) projected
  arc A2 (-47.8, 0) -> (-49.8, -2) centre (-47.8, -2) ccw projected
  line L6 (-49.8, -47.8) -> (-49.8, -2) projected
  arc A3 (-49.8, -47.8) -> (-47.8, -49.8) centre (-47.8, -47.8) ccw projected
  line L7 (-2, -49.8) -> (-47.8, -49.8) projected
  arc A4 (-2, -49.8) -> (0, -47.8) centre (-2, -47.8) ccw projected
  line L8 (0, -2) -> (0, -47.8) projected
  arc A5 (0, -2) -> (-2, 0) centre (-2, -2) ccw projected
  line L9 (-47.8, 0) -> (-2, 0) projected
  circle A6 centre (-39.35, -45.45) radius 2.4 projected
  circle A7 centre (-4.35, -39.35) radius 2.4 projected
  circle A8 centre (-45.45, -39.35) radius 2.4 projected
  circle A9 centre (-10.45, -45.45) radius 2.4 projected
  circle A10 centre (-4, -4) radius 1.75
  circle A11 centre (-45.8, -4) radius 1.75
  point P0 (0, 0)
  dimension "d182" = 3.5
  dimension "d183" = 3.5
  dimension "d184" = 4
  dimension "d185" = 4
  dimension "d186" = 4
  dimension "d187" = 4
  constraints: 2 centre point
  measures "d182" diameter of A10
  measures "d183" diameter of A11
  measures "d184" distance from line of A11.centre L9
  measures "d185" distance from line of L6 A11.centre
  measures "d186" distance from line of A10.centre L8
  measures "d187" distance from line of L9 A10.centre
extrude "Extrusion13" cut sketch "Skizze20" against normal through all contours A10 | A11
equation "\"d59\" = d58"
body "Solid1"
